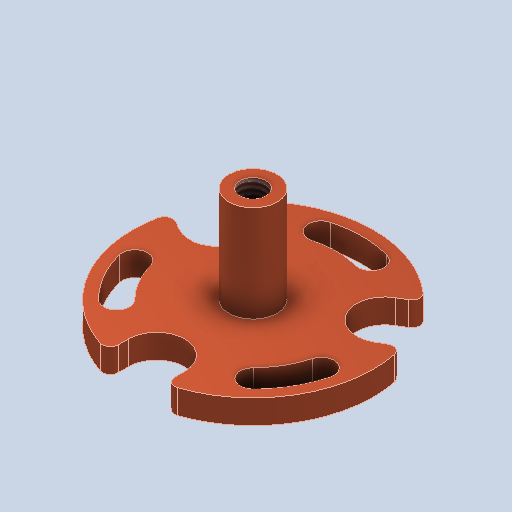
# Autodesk Inventor part: FrameSupport-Flange
Saved by Autodesk Inventor 2026 (Build 300175050, 175E)
## iProperties
Created: 2023-08-18
Part Number: FrameSupport-Flange
Material: Copper
Document SubType Name: Modeling
Designer: schanen
Density: 8.94 g/cm^3
Appearance: Copper - Satin
Author: schanen
Autodesk Inventor part; units mm, degrees
ref_plane "YZ Plane" through (0, 0, 0) normal (1, 0, 0) x (0, 1, 0)
ref_plane "XZ Plane" through (0, 0, 0) normal (0, 1, 0) x (-1, 0, 0)
ref_plane "XY Plane" through (0, 0, 0) normal (0, 0, 1) x (1, 0, 0)
sketch "Sketch1" plane through (0, 0, 0) normal (0, 1, 0) x (-1, 0, 0)
  circle A0 centre (0, 0) radius 15
  dimension "d0" = 30
  constraints: 1 centre point, 1 coincident
  measures "d0" diameter of A0
extrude "Extrusion1" add sketch "Sketch1" along normal blind 3
sketch "Sketch6" plane through (0, 3, 0) normal (0, 1, 0) x (1, 0, 0)
  circle A0 centre (0, 0) radius 3
  dimension "d24" = 6
  constraints: 1 centre point, 1 coincident
  measures "d24" diameter of A0
extrude "Extrusion4" add sketch "Sketch6" along normal blind 12
sketch "Sketch8" plane through (0, 15, 0) normal (0, 1, 0) x (1, 0, 0)
  point P0 (0, 0)
  point P1 (0, 0)
  constraints: 1 coincident
hole "Hole2" at (0, 15, 0) direction (0, -1, 0) diameter 3.242 end through all thread size "M4x0.7" class "6H" standard "ANSI Metric M Profile"
sketch "Sketch9" plane through (0, 3, 0) normal (0, 1, 0) x (1, 0, 0)
  arc A0 (3.1058, 11.5911) -> (-3.1058, 11.5911) centre (0, 0) ccw construction
  arc A1 (3.5199, 13.1366) -> (-3.5199, 13.1366) centre (0, 0) ccw
  arc A2 (2.6917, 10.0456) -> (-2.6917, 10.0456) centre (0, 0) ccw
  arc A3 (2.6917, 10.0456) -> (3.5199, 13.1366) centre (3.1058, 11.5911) ccw
  arc A4 (-3.5199, 13.1366) -> (-2.6917, 10.0456) centre (-3.1058, 11.5911) ccw
  circle A5 centre (0, 0) radius 15 projected
  point P0 (0, 15)
  dimension "d37" = 3.2
  dimension "d38" = 30
  dimension "d39" = 15
  dimension "d45" = 12
  constraints: 10 point on circle, 5 centre point, 4 tangent, 2 vertical alignment, 1 coincident, 1 other
  measures "d37" diameter of A3
  measures "d45" radius of A0
extrude "Extrusion6" cut sketch "Sketch9" against normal through all contours A3 A2 A4 A1
pattern_circular "Circular Pattern2" count 3 over 360 about axis through (0, 3, 0) along (0, 1, 0) of "Extrusion6"
sketch "Sketch11" plane through (0, 3, 0) normal (0, 1, 0) x (1, 0, 0)
  circle A0 centre (0, -12) radius 3.5
  line L0 (3.5, -12) -> (3.5, -14.586)
  line L1 (-3.5, -12) -> (-3.5, -14.586)
  arc A1 (-3.5, -14.586) -> (3.5, -14.586) centre (0, 0) ccw
  circle A2 centre (0, 0) radius 15 projected
  point P0 (-2.011, -14.8646)
  point P1 (2.011, -14.8646)
  dimension "d48" = 7
  dimension "d49" = 12
  constraints: 4 end point, 4 point on circle, 2 centre point, 2 tangent, 2 vertical, 1 coincident, 1 vertical alignment, 2 other
  measures "d48" diameter of A0
  measures "d49" distance of A0.centre point (0, 0)
extrude "Extrusion7" cut sketch "Sketch11" against normal through all contours A0 A1 | L0 A1 A0 | A0 A1 L1 | A0 A1
fillet "Fillet1" radius 1 2 edges at (-3.5, 1.5, 14.586) (3.5, 1.5, 14.586)
pattern_circular "Circular Pattern3" count 3 over 360 about axis through (0, 0, 0) along (0, 1, 0) of "Extrusion7", "Fillet1"
body "Solid1"
